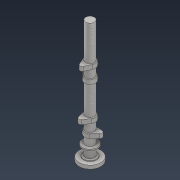
# Autodesk Inventor part: Wałek rozrządu
Saved by Autodesk Inventor 2022 (Build 260153000, 153)
## iProperties
Created: 2023-05-22
Part Number: Wałek rozrządu
Material: Generic
Document SubType Name: Modeling
Designer: wikto
Density: 1 g/cm^3
Appearance: Satin Brushed
Author: wikto
Autodesk Inventor part; units mm, degrees
ref_plane "YZ Plane" through (0, 0, 0) normal (1, 0, 0) x (0, 1, 0)
ref_plane "XZ Plane" through (0, 0, 0) normal (0, 1, 0) x (-1, 0, 0)
ref_plane "XY Plane" through (0, 0, 0) normal (0, 0, 1) x (1, 0, 0)
sketch "Sketch1" plane through (0, 0, 0) normal (0, 1, 0) x (-1, 0, 0)
  circle A0 centre (0, 0) radius 10
  dimension "d2" = 20
  constraints: 1 centre point, 1 coincident
  measures "d2" diameter of A0
extrude "Extrusion1" add sketch "Sketch1" along normal blind 283
ref_plane "Work Plane1" through (0, 181.485, 0) normal (0, 1, 0) x (1, 0, 0)
ref_plane "Work Plane2" through (0, 196.485, 0) normal (0, 1, 0) x (1, 0, 0)
ref_plane "Work Plane3" through (0, 166.485, 0) normal (0, 1, 0) x (1, 0, 0)
sketch "Sketch2" plane through (0, 196.485, 0) normal (0, 1, 0) x (1, 0, 0)
  circle A0 centre (0, 0) radius 12.5
  line L0 (-11.3632, -5.2083) -> (0, -30)
  line L1 (0, -30) -> (11.3632, -5.2083)
  dimension "d6" = 25
  dimension "d7" = 30
  constraints: 4 end point, 2 point on circle, 2 tangent, 1 centre point, 1 coincident, 1 vertical alignment
  measures "d6" diameter of A0
  measures "d7" distance of L0.end point (0, 0)
extrude "Extrusion2" add sketch "Sketch2" along normal mid plane 10
sketch "Sketch4" plane through (0, 166.485, 0) normal (0, 1, 0) x (1, 0, 0)
  circle A0 centre (0, 0) radius 12.5
  line L0 (0, -30) -> (11.3632, -5.2083) construction
  line L1 (0, 0) -> (0, -30) construction
  line L2 (0, 0) -> (-28.1908, 10.2606) construction
  line L3 (-1.0078, 12.4593) -> (-28.1908, 10.2606)
  line L4 (-28.1908, 10.2606) -> (-8.7807, -8.8966)
  point P0 (0, -12.5552)
  point P1 (0, -12.5)
  point P2 (6.0758, -7.9426)
  point P3 (10.4096, -7.2889)
  point P4 (0, -12.5552)
  dimension "d10" = 25
  dimension "d12" = 30
  dimension "d19" = 250
  constraints: 8 end point, 2 point on circle, 2 tangent, 1 centre point, 1 coincident, 1 vertical, 1 other
  measures "d10" diameter of A0
  measures "d12" distance of L1.start L2.end
extrude "Extrusion3" add sketch "Sketch4" along normal mid plane 10
ref_plane "Work Plane4" through (0, 72.715, 0) normal (0, 1, 0) x (1, 0, 0)
ref_plane "Work Plane5" through (0, 87.715, 0) normal (0, 1, 0) x (1, 0, 0)
ref_plane "Work Plane6" through (0, 57.715, 0) normal (0, 1, 0) x (1, 0, 0)
fillet "Fillet1" radius 5 2 edges at (-28.1908, 166.485, -10.2606) (0, 196.485, 30)
sketch "Sketch5" plane through (0, 87.715, 0) normal (0, 1, 0) x (1, 0, 0)
  circle A0 centre (0, 0) radius 12.5
  arc A1 (-4.5453, -20.0833) -> (4.5453, -20.0833) centre (0, -18) ccw projected
  line L0 (0, 0) -> (0, -18) construction
  line L1 (0, 0) -> (-5.2094, -29.5442) construction
  line L2 (-5.2094, -29.5442) -> (-12.095, -3.156)
  line L3 (-5.2094, -29.5442) -> (10.2862, -7.1024)
  dimension "d21" = 25
  dimension "d22" = 10
  dimension "d23" = 30
  constraints: 8 end point, 2 point on circle, 2 tangent, 1 centre point, 1 coincident, 1 vertical
  measures "d21" diameter of A0
  measures "d22" angle of L1 L0
  measures "d23" distance of L0.start L1.end
extrude "Extrusion4" add sketch "Sketch5" along normal mid plane 10
sketch "Sketch6" plane through (0, 57.715, 0) normal (0, 1, 0) x (1, 0, 0)
  circle A0 centre (0, 0) radius 12.5
  line L0 (-8.7807, -8.8966) -> (-20.4267, 2.5977) projected
  line L1 (8.7807, -8.8966) -> (28.1908, 10.2606)
  line L2 (28.1908, 10.2606) -> (1.0078, 12.4593)
  line L3 (0, 0) -> (0, -18) construction
  line L4 (28.1908, 10.2606) -> (0, 0) construction
  dimension "d26" = 25
  dimension "d27" = 18
  dimension "d28" = 30
  dimension "d29" = 250
  constraints: 8 end point, 2 point on circle, 2 tangent, 1 centre point, 1 coincident, 1 vertical
  measures "d26" diameter of A0
  measures "d27" distance of L3.start L3.end
  measures "d28" distance of L1.end L3.start
extrude "Extrusion5" add sketch "Sketch6" along normal mid plane 10
fillet "Fillet2" radius 5 2 edges at (28.1908, 57.715, -10.2606) (-5.2094, 87.715, 29.5442)
sketch "Sketch7" plane through (0, 0, 0) normal (0, -1, 0) x (1, 0, 0)
  circle A0 centre (0, 0) radius 15
  circle A1 centre (0, 0) radius 25
  dimension "d33" = 30
  dimension "d34" = 50
  constraints: 2 centre point, 2 coincident
  measures "d33" diameter of A0
  measures "d34" diameter of A1
extrude "Extrusion6" add sketch "Sketch7" against normal blind 8
extrude "Extrusion7" add sketch "Sketch7" against normal blind 10 contours A0
sketch "Sketch8" plane through (0, 0, 0) normal (0, -1, 0) x (1, 0, 0)
  line L0 (15, -2.5) -> (-15, -2.5)
  line L1 (-15, -2.5) -> (-15, 2.5)
  line L2 (-15, 2.5) -> (15, 2.5)
  line L3 (15, 2.5) -> (15, -2.5)
  line L4 (15, -2.5) -> (-15, 2.5) construction
  line L5 (-15, -2.5) -> (15, 2.5) construction
  circle A0 centre (0, 0) radius 20
  circle A1 centre (0, 0) radius 5
  point P0 (-20, 0)
  point P1 (10, -17.3205)
  point P2 (10, 17.3205)
  point P3 (4.3301, 2.5)
  point P4 (-4.3301, 2.5)
  point P5 (-4.3301, -2.5)
  point P6 (4.3301, -2.5)
  dimension "d43" = 40
  dimension "d41" = 360
  dimension "d44" = 5
  dimension "d45" = 30
  dimension "d48" = 10
  constraints: 12 end point, 3 midpoint, 2 coincident, 2 horizontal alignment, 2 parallel, 1 centre point, 1 horizontal, 1 perpendicular, 6 other
  measures "d44" distance between parallel lines of L0 L2
  measures "d45" distance between parallel lines of L1 L3
  measures "d48" diameter of A1
extrude "Extrusion8" cut sketch "Sketch8" against normal blind 5 contours L0 A1 L2 L3 | A1 L0 | L0 A1 L2 | L0 L1 L2 A1 | L2 A1
hole "Hole1" at (-20, 0, 0) at (10, 0, -17.3205) at (10, 0, 17.3205) direction (0, 1, 0) diameter 4.134 depth 5 thread size "M5x0.8" class "6H" standard "ISO Metric profile"
ref_plane "Work Plane7" through (0, 31.76, 0) normal (0, 1, 0) x (1, 0, 0)
sketch "Sketch9" plane through (0, 31.76, 0) normal (0, 1, 0) x (1, 0, 0)
  circle A0 centre (0, 0) radius 17.5
  dimension "d57" = 35
  constraints: 1 centre point, 1 coincident
  measures "d57" diameter of A0
extrude "Extrusion9" add sketch "Sketch9" along normal blind 3
body "Solid1"
